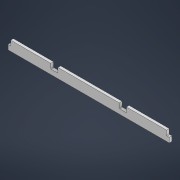
# Autodesk Inventor part: Length Board
Saved by Autodesk Inventor 2021 (Build 250183000, 183)
## iProperties
Created: 2021-03-26
Part Number: Length Board
Material: Generic
Document SubType Name: Modeling
Designer: allen
Density: 1 g/cm^3
Appearance: Default
Author: allen
Autodesk Inventor part; units mm, degrees
sketch "Sketch1" plane through (0, 0, 0) normal (0, 0, 1) x (1, 0, 0)
  line L0 (0, 0) -> (910, 0)
  line L1 (910, 0) -> (910, 55)
  line L2 (910, 55) -> (0, 55)
  line L3 (0, 55) -> (0, 0)
  dimension "d0" = 910
  dimension "d1" = 55
  constraints: 8 end point, 2 parallel, 1 horizontal, 1 perpendicular
  measures "d0" distance of L0.start L0.end
  measures "d1" distance of L2.end L0.start
extrude "Extrusion1" add sketch "Sketch1" along normal blind 15
ref_plane "Work Plane1" through (455, 0, 0) normal (-1, 0, 0) x (0, 0, 1)
sketch "Sketch3" plane through (0, 0, 15) normal (0, 0, 1) x (1, 0, 0)
  line L0 (910, 55) -> (0, 55) projected
  line L1 (0, 55) -> (15, 55)
  line L2 (15, 55) -> (15, 27.5)
  line L3 (15, 27.5) -> (0, 27.5)
  line L4 (0, 27.5) -> (0, 55)
  line L5 (241.667, 55) -> (281.667, 55)
  line L6 (281.667, 55) -> (281.667, 27.5)
  line L7 (281.667, 27.5) -> (241.667, 27.5)
  line L8 (241.667, 27.5) -> (241.667, 55)
  line L9 (455, 55) -> (455, 32.488)
  line L10 (910, 55) -> (895, 55)
  line L11 (895, 55) -> (895, 27.5)
  line L12 (895, 27.5) -> (910, 27.5)
  line L13 (910, 27.5) -> (910, 55)
  line L14 (668.333, 55) -> (628.333, 55)
  line L15 (628.333, 55) -> (628.333, 27.5)
  line L16 (628.333, 27.5) -> (668.333, 27.5)
  line L17 (668.333, 27.5) -> (668.333, 55)
  point P0 (0, 0)
  point P1 (910, 0)
  point P2 (668.333, 55)
  point P3 (628.333, 55)
  dimension "d12" = 15
  dimension "d13" = 27.5
  dimension "d14" = 226.667
  dimension "d15" = 40
  constraints: 34 end point, 8 symmetric about line, 4 parallel, 2 horizontal, 2 perpendicular, 1 collinear, 1 midpoint, 1 point on line, 1 vertical
  measures "d12" distance of L2.end L3.end
  measures "d13" distance of L3.end L0.end
  measures "d14" distance between parallel lines of L8 L2
  measures "d15" distance of L6.end L7.end
extrude "Extrusion2" cut sketch "Sketch3" against normal through all
ref_plane "Work Plane2" through (455, 0, 0) normal (-1, 0, 0) x (0, 0, 1)
ref_plane "Work Plane3" through (0, 0, 7.5) normal (0, 0, 1) x (1, 0, 0)
fillet "Fillet1" radius 3 6 edges at (895, 27.5, 7.5) (668.333, 27.5, 7.5) (628.333, 27.5, 7.5) (281.667, 27.5, 7.5) (241.667, 27.5, 7.5) (15, 27.5, 7.5)
body "Solid1"
